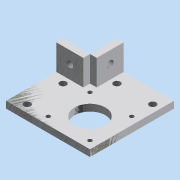
# Autodesk Inventor part: Motor Mount
Saved by Autodesk Inventor 2015 (Build 190159000, 159)
## iProperties
Created: 2016-09-07
Part Number: Motor Mount
Material: Generic
Document SubType Name: Modeling
Designer: Dustin
Density: 1 g/cm^3
Appearance: Default
Author: Dustin
Autodesk Inventor part; units mm, degrees
ref_plane "YZ Plane" through (0, 0, 0) normal (1, 0, 0) x (0, 1, 0)
ref_plane "XZ Plane" through (0, 0, 0) normal (0, 1, 0) x (-1, 0, 0)
ref_plane "XY Plane" through (0, 0, 0) normal (0, 0, 1) x (1, 0, 0)
sketch "Sketch1" plane through (0, 0, 0) normal (0, 0, 1) x (1, 0, 0)
  line L0 (0, 0) -> (42.3, 0)
  line L1 (42.3, 0) -> (42.3, 42.3)
  line L2 (42.3, 42.3) -> (0, 42.3)
  line L3 (0, 42.3) -> (0, 0)
  circle A0 centre (21.15, 21.15) radius 11.5
  line L4 (0, 0.3) -> (0, 42.3)
  line L5 (0, 42.3) -> (42.3, 42.3)
  line L6 (0, 42.3) -> (42.3, 42.3)
  line L7 (42.3, 42.3) -> (42.3, 62.3)
  line L8 (42.3, 62.3) -> (0, 62.3)
  line L9 (0, 62.3) -> (0, 42.3)
  line L10 (0, 42.3) -> (-20, 42.3)
  line L11 (-20, 42.3) -> (-20, 0)
  line L12 (-20, 0) -> (0, 0)
  line L13 (0, 0) -> (0, 42.3)
  point P0 (5.65, 36.65)
  point P1 (36.65, 36.65)
  point P2 (36.65, 5.65)
  point P3 (5.65, 5.65)
  point P4 (10, 52.3)
  point P5 (36.65, 52.3)
  point P6 (-10, 32.3)
  point P7 (-10, 5.65)
  dimension "d0" = 42.3
  dimension "d1" = 23
  dimension "d2" = 31
  dimension "d3" = 31
  dimension "d4" = 31
  dimension "d8" = 31
  dimension "d12" = 21.15
  dimension "d16" = 42.3
  dimension "d17" = 5.65
  dimension "d18" = 5.65
  dimension "d19" = 5.65
  dimension "d20" = 5.65
  dimension "d21" = 20
  dimension "d22" = 20
  dimension "d39" = 21.15
  dimension "d42" = 10
  dimension "d43" = 10
  constraints: 28 end point, 6 parallel, 4 horizontal, 3 perpendicular, 1 centre point
  measures "d0" distance of L1.end L2.end
  measures "d1" diameter of A0
  measures "d2" distance of point (36.65, 36.65) point (5.65, 36.65)
  measures "d3" distance of point (5.65, 5.65) point (5.65, 36.65)
  measures "d4" distance of point (36.65, 5.65) point (5.65, 5.65)
  measures "d8" distance of point (36.65, 5.65) point (36.65, 36.65)
  measures "d12" distance from line of A0.centre L3
  measures "d16" distance of L2.end L0.start
  measures "d17" distance from line of L3 point (5.65, 36.65)
  measures "d18" distance from line of L2 point (36.65, 36.65)
  measures "d19" distance from line of L1 point (36.65, 5.65)
  measures "d20" distance from line of L0 point (5.65, 5.65)
  measures "d21" distance of L6.end L7.end
  measures "d22" distance of L2.end L10.end
  measures "d39" distance from line of L5 A0.centre
  measures "d42" distance from line of L9 point (10, 52.3)
  measures "d43" distance from line of L10 point (-10, 32.3)
extrude "Extrusion1" add sketch "Sketch1" along normal blind 5
hole "Hole1" at (5.65, 36.65, 0) at (36.65, 36.65, 0) at (36.65, 5.65, 0) at (5.65, 5.65, 0) direction (0, 0, 1) diameter 3 depth 8 tip angle 118
hole "Hole2" at (10, 52.3, 0) at (36.65, 52.3, 0) at (-10, 32.3, 0) at (-10, 5.65, 0) direction (0, 0, 1) diameter 5 depth 8 tip angle 118
sketch "Sketch3" plane through (0, 0, 5) normal (0, 0, 1) x (1, 0, 0)
  line L0 (-20, 42.3) -> (0, 42.3)
  line L1 (0, 42.3) -> (0, 37.3)
  line L2 (0, 37.3) -> (-20, 37.3)
  line L3 (-20, 37.3) -> (-20, 42.3)
  line L4 (0, 62.3) -> (5, 62.3)
  line L5 (5, 62.3) -> (5, 42.3)
  line L6 (5, 42.3) -> (0, 42.3)
  line L7 (0, 42.3) -> (0, 62.3)
  point P0 (0, 0)
  dimension "d40" = 5
  dimension "d41" = 5
  constraints: 16 end point, 4 parallel, 2 horizontal, 2 perpendicular, 1 point on line
  measures "d40" distance of L2.end L0.start
  measures "d41" distance of L4.start L4.end
extrude "Extrusion2" add sketch "Sketch3" along normal blind 19
sketch "Sketch4" plane through (-20, 37.3, 5) normal (0, -1, 0) x (1, 0, 0)
  line L0 (0, 0) -> (62.3, 0) projected
  line L1 (0, 0) -> (0, 19) projected
  line L2 (0, 19) -> (20, 19) projected
  point P0 (20, -5)
  point P1 (10, 10)
  dimension "d46" = 10
  dimension "d47" = 10
  measures "d46" distance from line of L0 point (10, 10)
  measures "d47" distance from line of L1 point (10, 10)
hole "Hole3" at (-10, 37.3, 15) direction (0, 1, 0) diameter 5 depth 8 tip angle 118
sketch "Sketch5" plane through (5, 42.3, 5) normal (1, 0, 0) x (0, 0, -1)
  line L0 (-19, 0) -> (-19, 20) projected
  line L1 (0, -42.3) -> (0, 20) projected
  line L2 (0, 20) -> (-19, 20) projected
  point P0 (5, -42.3)
  point P1 (-10, 10)
  dimension "d58" = 10
  dimension "d59" = 10
  measures "d58" distance from line of L1 point (-10, 10)
  measures "d59" distance from line of L2 point (-10, 10)
hole "Hole4" at (5, 52.3, 15) direction (-1, 0, 0) diameter 5 depth 8 tip angle 118
body "Solid1"
